Autodesk Fusion 360 part; units mm, degrees
(part 2 of 3)
extrude "Estrusione_Slitta_SG90_Sinistra_guida_01" add sketch "Schizzo30 (2)" along normal blind 23.5 bodies 11 in component "04_Torretta_parte_fissa_azimut"
ref_plane "Piano di lavoro17" through (-63.5, 0, 0) normal (1, 0, 0) x (0, 1, 0) in component "04_Torretta_parte_fissa_azimut"
sketch "Schizzo31 (2)" plane through (-63.5, 0, 0) normal (1, 0, 0) x (0, 0, -1) in component "04_Torretta_parte_fissa_azimut"
  line L0 (-74.9, 11) -> (-88.1, 11)
  line L1 (-88.1, 11) -> (-88.1, 13.5)
  line L2 (-88.1, 13.5) -> (-74.9, 13.5)
  line L3 (-74.9, 13.5) -> (-74.9, 11)
extrude "Estrusione_Slitta_SG90_Sinistra_guida_02" add sketch "Schizzo31 (2)" along normal blind 23.5 bodies 11 in component "04_Torretta_parte_fissa_azimut"
ref_plane "Piano di lavoro18" through (-63.5, 0, 0) normal (1, 0, 0) x (0, 1, 0) in component "04_Torretta_parte_fissa_azimut"
sketch "Schizzo32 (2)" plane through (-63.5, 0, 0) normal (1, 0, 0) x (0, 0, -1) in component "04_Torretta_parte_fissa_azimut"
  circle A0 centre (-81.5, -23.55) radius 1.1
extrude "Preforo_M2_5_slitta_Sinistra_01" cut sketch "Schizzo32 (2)" along normal blind 23.5 bodies 11 in component "04_Torretta_parte_fissa_azimut"
ref_plane "Piano di lavoro19" through (-63.5, 0, 0) normal (1, 0, 0) x (0, 1, 0) in component "04_Torretta_parte_fissa_azimut"
sketch "Schizzo33 (2)" plane through (-63.5, 0, 0) normal (1, 0, 0) x (0, 0, -1) in component "04_Torretta_parte_fissa_azimut"
  circle A0 centre (-81.5, 12.25) radius 1.1
extrude "Preforo_M2_5_slitta_Sinistra_02" cut sketch "Schizzo33 (2)" along normal blind 23.5 bodies 11 in component "04_Torretta_parte_fissa_azimut"
ref_plane "Piano di lavoro20" through (0, 0, 72.4) normal (0, 0, 1) x (1, 0, 0) in component "04_Torretta_parte_fissa_azimut"
sketch "Schizzo34 (2)" plane through (0, 0, 72.4) normal (0, 0, 1) x (1, 0, 0) in component "04_Torretta_parte_fissa_azimut"
  line L0 (40, -24.8) -> (63.5, -24.8)
  line L1 (63.5, -24.8) -> (63.5, 13.5)
  line L2 (63.5, 13.5) -> (40, 13.5)
  line L3 (40, 13.5) -> (40, -24.8)
extrude "Estrusione_Slitta_SG90_Destra_ripiano_Inferiore" add sketch "Schizzo34 (2)" along normal blind 2.5 bodies 11 in component "04_Torretta_parte_fissa_azimut"
ref_plane "Piano di lavoro21" through (0, 0, 88.1) normal (0, 0, 1) x (1, 0, 0) in component "04_Torretta_parte_fissa_azimut"
sketch "Schizzo35 (2)" plane through (0, 0, 88.1) normal (0, 0, 1) x (1, 0, 0) in component "04_Torretta_parte_fissa_azimut"
  line L0 (40, -24.8) -> (63.5, -24.8)
  line L1 (63.5, -24.8) -> (63.5, 13.5)
  line L2 (63.5, 13.5) -> (40, 13.5)
  line L3 (40, 13.5) -> (40, -24.8)
extrude "Estrusione_Slitta_SG90_Destra_ripiano_Superiore" add sketch "Schizzo35 (2)" along normal blind 2.5 bodies 11 in component "04_Torretta_parte_fissa_azimut"
ref_plane "Piano di lavoro22" through (0, 0, 72.4) normal (0, 0, 1) x (1, 0, 0) in component "04_Torretta_parte_fissa_azimut"
sketch "Schizzo36 (2)" plane through (0, 0, 72.4) normal (0, 0, 1) x (1, 0, 0) in component "04_Torretta_parte_fissa_azimut"
  line L0 (61.5, -8.15) -> (63.5, -8.15)
  line L1 (63.5, -8.15) -> (63.5, -3.15)
  line L2 (63.5, -3.15) -> (61.5, -3.15)
  line L3 (61.5, -3.15) -> (61.5, -8.15)
extrude "Uscita_cavo_5x2_SG90_Destra" cut sketch "Schizzo36 (2)" along normal blind 2.5 bodies 11 in component "04_Torretta_parte_fissa_azimut"
ref_plane "Piano di lavoro23" through (40, 0, 0) normal (1, 0, 0) x (0, 1, 0) in component "04_Torretta_parte_fissa_azimut"
sketch "Schizzo37 (2)" plane through (40, 0, 0) normal (1, 0, 0) x (0, 0, -1) in component "04_Torretta_parte_fissa_azimut"
  line L0 (-74.9, -24.8) -> (-88.1, -24.8)
  line L1 (-88.1, -24.8) -> (-88.1, -22.3)
  line L2 (-88.1, -22.3) -> (-74.9, -22.3)
  line L3 (-74.9, -22.3) -> (-74.9, -24.8)
extrude "Estrusione_Slitta_SG90_Destra_guida_01" add sketch "Schizzo37 (2)" along normal blind 23.5 bodies 11 in component "04_Torretta_parte_fissa_azimut"
ref_plane "Piano di lavoro24" through (40, 0, 0) normal (1, 0, 0) x (0, 1, 0) in component "04_Torretta_parte_fissa_azimut"
sketch "Schizzo38 (2)" plane through (40, 0, 0) normal (1, 0, 0) x (0, 0, -1) in component "04_Torretta_parte_fissa_azimut"
  line L0 (-74.9, 11) -> (-88.1, 11)
  line L1 (-88.1, 11) -> (-88.1, 13.5)
  line L2 (-88.1, 13.5) -> (-74.9, 13.5)
  line L3 (-74.9, 13.5) -> (-74.9, 11)
extrude "Estrusione_Slitta_SG90_Destra_guida_02" add sketch "Schizzo38 (2)" along normal blind 23.5 bodies 11 in component "04_Torretta_parte_fissa_azimut"
ref_plane "Piano di lavoro25" through (40, 0, 0) normal (1, 0, 0) x (0, 1, 0) in component "04_Torretta_parte_fissa_azimut"
sketch "Schizzo39 (2)" plane through (40, 0, 0) normal (1, 0, 0) x (0, 0, -1) in component "04_Torretta_parte_fissa_azimut"
  circle A0 centre (-81.5, -23.55) radius 1.1
extrude "Preforo_M2_5_slitta_Destra_01" cut sketch "Schizzo39 (2)" along normal blind 23.5 bodies 11 in component "04_Torretta_parte_fissa_azimut"
ref_plane "Piano di lavoro26" through (40, 0, 0) normal (1, 0, 0) x (0, 1, 0) in component "04_Torretta_parte_fissa_azimut"
sketch "Schizzo40 (2)" plane through (40, 0, 0) normal (1, 0, 0) x (0, 0, -1) in component "04_Torretta_parte_fissa_azimut"
  circle A0 centre (-81.5, 12.25) radius 1.1
extrude "Preforo_M2_5_slitta_Destra_02" cut sketch "Schizzo40 (2)" along normal blind 23.5 bodies 11 in component "04_Torretta_parte_fissa_azimut"
ref_plane "Piano di lavoro1" through (-63, 0, 0) normal (1, 0, 0) x (0, 1, 0) in component "05_Servo_TowerPro_SG90_Sinistro_statore_riferimento"
sketch "Schizzo1 (11)" plane through (-63, 0, 0) normal (1, 0, 0) x (0, 0, -1) in component "05_Servo_TowerPro_SG90_Sinistro_statore_riferimento"
  line L0 (-75.4, -17) -> (-87.6, -17)
  line L1 (-87.6, -17) -> (-87.6, 5.7)
  line L2 (-87.6, 5.7) -> (-75.4, 5.7)
  line L3 (-75.4, 5.7) -> (-75.4, -17)
extrude "Estrusione_Corpo_SG90_Sinistro" add sketch "Schizzo1 (11)" along normal blind 27 separate body makes body 12 in component "05_Servo_TowerPro_SG90_Sinistro_statore_riferimento"
ref_plane "Piano di lavoro2" through (-42, 0, 0) normal (1, 0, 0) x (0, 1, 0) in component "05_Servo_TowerPro_SG90_Sinistro_statore_riferimento"
sketch "Schizzo2 (10)" plane through (-42, 0, 0) normal (1, 0, 0) x (0, 0, -1) in component "05_Servo_TowerPro_SG90_Sinistro_statore_riferimento"
  line L0 (-75.4, -21.8) -> (-87.6, -21.8)
  line L1 (-87.6, -21.8) -> (-87.6, 10.5)
  line L2 (-87.6, 10.5) -> (-75.4, 10.5)
  line L3 (-75.4, 10.5) -> (-75.4, -21.8)
extrude "Estrusione_Alette_fissaggio_reali_SG90_Sinistro" add sketch "Schizzo2 (10)" along normal blind 2 bodies 12 in component "05_Servo_TowerPro_SG90_Sinistro_statore_riferimento"
ref_plane "Piano di lavoro3" through (-42, 0, 0) normal (1, 0, 0) x (0, 1, 0) in component "05_Servo_TowerPro_SG90_Sinistro_statore_riferimento"
sketch "Schizzo3 (9)" plane through (-42, 0, 0) normal (1, 0, 0) x (0, 0, -1) in component "05_Servo_TowerPro_SG90_Sinistro_statore_riferimento"
  circle A0 centre (-81.5, -20.05) radius 1.25
extrude "Foro_M2_5_aletta_reale_Sinistro_01" cut sketch "Schizzo3 (9)" along normal blind 2 bodies 12 in component "05_Servo_TowerPro_SG90_Sinistro_statore_riferimento"
ref_plane "Piano di lavoro4" through (-42, 0, 0) normal (1, 0, 0) x (0, 1, 0) in component "05_Servo_TowerPro_SG90_Sinistro_statore_riferimento"
sketch "Schizzo4 (8)" plane through (-42, 0, 0) normal (1, 0, 0) x (0, 0, -1) in component "05_Servo_TowerPro_SG90_Sinistro_statore_riferimento"
  circle A0 centre (-81.5, 8.75) radius 1.25
extrude "Foro_M2_5_aletta_reale_Sinistro_02" cut sketch "Schizzo4 (8)" along normal blind 2 bodies 12 in component "05_Servo_TowerPro_SG90_Sinistro_statore_riferimento"
ref_plane "Piano di lavoro1" through (36, 0, 0) normal (1, 0, 0) x (0, 1, 0) in component "06_Servo_TowerPro_SG90_Destro_statore_riferimento"
sketch "Schizzo1 (12)" plane through (36, 0, 0) normal (1, 0, 0) x (0, 0, -1) in component "06_Servo_TowerPro_SG90_Destro_statore_riferimento"
  line L0 (-75.4, -17) -> (-87.6, -17)
  line L1 (-87.6, -17) -> (-87.6, 5.7)
  line L2 (-87.6, 5.7) -> (-75.4, 5.7)
  line L3 (-75.4, 5.7) -> (-75.4, -17)
extrude "Estrusione_Corpo_SG90_Destro" add sketch "Schizzo1 (12)" along normal blind 27 separate body makes body 13 in component "06_Servo_TowerPro_SG90_Destro_statore_riferimento"
ref_plane "Piano di lavoro2" through (40, 0, 0) normal (1, 0, 0) x (0, 1, 0) in component "06_Servo_TowerPro_SG90_Destro_statore_riferimento"
sketch "Schizzo2 (11)" plane through (40, 0, 0) normal (1, 0, 0) x (0, 0, -1) in component "06_Servo_TowerPro_SG90_Destro_statore_riferimento"
  line L0 (-75.4, -21.8) -> (-87.6, -21.8)
  line L1 (-87.6, -21.8) -> (-87.6, 10.5)
  line L2 (-87.6, 10.5) -> (-75.4, 10.5)
  line L3 (-75.4, 10.5) -> (-75.4, -21.8)
extrude "Estrusione_Alette_fissaggio_reali_SG90_Destro" add sketch "Schizzo2 (11)" along normal blind 2 bodies 13 in component "06_Servo_TowerPro_SG90_Destro_statore_riferimento"
ref_plane "Piano di lavoro3" through (40, 0, 0) normal (1, 0, 0) x (0, 1, 0) in component "06_Servo_TowerPro_SG90_Destro_statore_riferimento"
sketch "Schizzo3 (10)" plane through (40, 0, 0) normal (1, 0, 0) x (0, 0, -1) in component "06_Servo_TowerPro_SG90_Destro_statore_riferimento"
  circle A0 centre (-81.5, -20.05) radius 1.25
extrude "Foro_M2_5_aletta_reale_Destro_01" cut sketch "Schizzo3 (10)" along normal blind 2 bodies 13 in component "06_Servo_TowerPro_SG90_Destro_statore_riferimento"
ref_plane "Piano di lavoro4" through (40, 0, 0) normal (1, 0, 0) x (0, 1, 0) in component "06_Servo_TowerPro_SG90_Destro_statore_riferimento"
sketch "Schizzo4 (9)" plane through (40, 0, 0) normal (1, 0, 0) x (0, 0, -1) in component "06_Servo_TowerPro_SG90_Destro_statore_riferimento"
  circle A0 centre (-81.5, 8.75) radius 1.25
extrude "Foro_M2_5_aletta_reale_Destro_02" cut sketch "Schizzo4 (9)" along normal blind 2 bodies 13 in component "06_Servo_TowerPro_SG90_Destro_statore_riferimento"
ref_plane "Piano di lavoro1" through (0, 0, 79.5) normal (0, 0, 1) x (1, 0, 0) in component "09_Torretta_parte_mobile_elevazione"
sketch "Schizzo1 (13)" plane through (0, 0, 79.5) normal (0, 0, 1) x (1, 0, 0) in component "09_Torretta_parte_mobile_elevazione"
  line L0 (-27, -20) -> (27, -20)
  line L1 (27, -20) -> (27, 50)
  line L2 (27, 50) -> (-27, 50)
  line L3 (-27, 50) -> (-27, -20)
extrude "Estrusione_Piastra_culla_mobile" add sketch "Schizzo1 (13)" along normal blind 4 separate body makes body 14 in component "09_Torretta_parte_mobile_elevazione"
sketch "Schizzo2 (12)" plane through (0, 0, 79.5) normal (0, 0, 1) x (1, 0, 0) in component "09_Torretta_parte_mobile_elevazione"
  line L0 (-3, -17) -> (3, -17)
  line L1 (3, -17) -> (3, -13)
  line L2 (3, -13) -> (-3, -13)
  line L3 (-3, -13) -> (-3, -17)
extrude "Passaggio_6x4_connettore_cannone_sotto_culla" cut sketch "Schizzo2 (12)" along normal blind 4 bodies 14 in component "09_Torretta_parte_mobile_elevazione"
sketch "Schizzo3 (11)" plane through (0, 0, 79.5) normal (0, 0, 1) x (1, 0, 0) in component "09_Torretta_parte_mobile_elevazione"
  line L0 (-7, -17.5) -> (-5, -17.5)
  line L1 (-5, -17.5) -> (-5, -12.5)
  line L2 (-5, -12.5) -> (-7, -12.5)
  line L3 (-7, -12.5) -> (-7, -17.5)
extrude "Asola_fascetta_ansa_cannone_mobile_01" cut sketch "Schizzo3 (11)" along normal blind 4 bodies 14 in component "09_Torretta_parte_mobile_elevazione"
sketch "Schizzo4 (10)" plane through (0, 0, 79.5) normal (0, 0, 1) x (1, 0, 0) in component "09_Torretta_parte_mobile_elevazione"
  line L0 (5, -17.5) -> (7, -17.5)
  line L1 (7, -17.5) -> (7, -12.5)
  line L2 (7, -12.5) -> (5, -12.5)
  line L3 (5, -12.5) -> (5, -17.5)
extrude "Asola_fascetta_ansa_cannone_mobile_02" cut sketch "Schizzo4 (10)" along normal blind 4 bodies 14 in component "09_Torretta_parte_mobile_elevazione"
sketch "Schizzo5 (4)" plane through (0, 0, 79.5) normal (0, 0, 1) x (1, 0, 0) in component "09_Torretta_parte_mobile_elevazione"
  circle A0 centre (-20, -5) radius 1.75
extrude "Foro_fissaggio_PCB_cannone_01" cut sketch "Schizzo5 (4)" along normal blind 4 bodies 14 in component "09_Torretta_parte_mobile_elevazione"
sketch "Schizzo6 (4)" plane through (0, 0, 79.5) normal (0, 0, 1) x (1, 0, 0) in component "09_Torretta_parte_mobile_elevazione"
  line L0 (-17.1, -3.3257) -> (-20, -1.6514)
  line L1 (-20, -1.6514) -> (-22.9, -3.3257)
  line L2 (-22.9, -3.3257) -> (-22.9, -6.6743)
  line L3 (-22.9, -6.6743) -> (-20, -8.3486)
  line L4 (-20, -8.3486) -> (-17.1, -6.6743)
  line L5 (-17.1, -6.6743) -> (-17.1, -3.3257)
extrude "Sede_dado_M3_PCB_cannone_01" cut sketch "Schizzo6 (4)" along normal blind 2.6 bodies 14 in component "09_Torretta_parte_mobile_elevazione"
sketch "Schizzo7 (4)" plane through (0, 0, 79.5) normal (0, 0, 1) x (1, 0, 0) in component "09_Torretta_parte_mobile_elevazione"
  circle A0 centre (20, -5) radius 1.75
extrude "Foro_fissaggio_PCB_cannone_02" cut sketch "Schizzo7 (4)" along normal blind 4 bodies 14 in component "09_Torretta_parte_mobile_elevazione"
sketch "Schizzo8 (4)" plane through (0, 0, 79.5) normal (0, 0, 1) x (1, 0, 0) in component "09_Torretta_parte_mobile_elevazione"
  line L0 (22.9, -3.3257) -> (20, -1.6514)
  line L1 (20, -1.6514) -> (17.1, -3.3257)
  line L2 (17.1, -3.3257) -> (17.1, -6.6743)
  line L3 (17.1, -6.6743) -> (20, -8.3486)
  line L4 (20, -8.3486) -> (22.9, -6.6743)
  line L5 (22.9, -6.6743) -> (22.9, -3.3257)
extrude "Sede_dado_M3_PCB_cannone_02" cut sketch "Schizzo8 (4)" along normal blind 2.6 bodies 14 in component "09_Torretta_parte_mobile_elevazione"
sketch "Schizzo9 (4)" plane through (0, 0, 79.5) normal (0, 0, 1) x (1, 0, 0) in component "09_Torretta_parte_mobile_elevazione"
  circle A0 centre (-20, 35) radius 1.75
extrude "Foro_fissaggio_PCB_cannone_03" cut sketch "Schizzo9 (4)" along normal blind 4 bodies 14 in component "09_Torretta_parte_mobile_elevazione"
sketch "Schizzo10 (4)" plane through (0, 0, 79.5) normal (0, 0, 1) x (1, 0, 0) in component "09_Torretta_parte_mobile_elevazione"
  line L0 (-17.1, 36.6743) -> (-20, 38.3486)
  line L1 (-20, 38.3486) -> (-22.9, 36.6743)
  line L2 (-22.9, 36.6743) -> (-22.9, 33.3257)
  line L3 (-22.9, 33.3257) -> (-20, 31.6514)
  line L4 (-20, 31.6514) -> (-17.1, 33.3257)
  line L5 (-17.1, 33.3257) -> (-17.1, 36.6743)
extrude "Sede_dado_M3_PCB_cannone_03" cut sketch "Schizzo10 (4)" along normal blind 2.6 bodies 14 in component "09_Torretta_parte_mobile_elevazione"
sketch "Schizzo11 (4)" plane through (0, 0, 79.5) normal (0, 0, 1) x (1, 0, 0) in component "09_Torretta_parte_mobile_elevazione"
  circle A0 centre (20, 35) radius 1.75
extrude "Foro_fissaggio_PCB_cannone_04" cut sketch "Schizzo11 (4)" along normal blind 4 bodies 14 in component "09_Torretta_parte_mobile_elevazione"
sketch "Schizzo12 (4)" plane through (0, 0, 79.5) normal (0, 0, 1) x (1, 0, 0) in component "09_Torretta_parte_mobile_elevazione"
  line L0 (22.9, 36.6743) -> (20, 38.3486)
  line L1 (20, 38.3486) -> (17.1, 36.6743)
  line L2 (17.1, 36.6743) -> (17.1, 33.3257)
  line L3 (17.1, 33.3257) -> (20, 31.6514)
  line L4 (20, 31.6514) -> (22.9, 33.3257)
  line L5 (22.9, 33.3257) -> (22.9, 36.6743)
extrude "Sede_dado_M3_PCB_cannone_04" cut sketch "Schizzo12 (4)" along normal blind 2.6 bodies 14 in component "09_Torretta_parte_mobile_elevazione"
sketch "Schizzo13 (4)" plane through (0, 0, 79.5) normal (0, 0, 1) x (1, 0, 0) in component "09_Torretta_parte_mobile_elevazione"
  circle A0 centre (-22.5, -10) radius 1.1
extrude "Preforo_cieco_guancia_cornetto_Sinistra_01" cut sketch "Schizzo13 (4)" along normal blind 3 bodies 14 in component "09_Torretta_parte_mobile_elevazione"
sketch "Schizzo14 (4)" plane through (0, 0, 79.5) normal (0, 0, 1) x (1, 0, 0) in component "09_Torretta_parte_mobile_elevazione"
  circle A0 centre (-22.5, 10) radius 1.1
extrude "Preforo_cieco_guancia_cornetto_Sinistra_02" cut sketch "Schizzo14 (4)" along normal blind 3 bodies 14 in component "09_Torretta_parte_mobile_elevazione"
sketch "Schizzo15 (4)" plane through (0, 0, 79.5) normal (0, 0, 1) x (1, 0, 0) in component "09_Torretta_parte_mobile_elevazione"
  circle A0 centre (22.5, -10) radius 1.1
extrude "Preforo_cieco_guancia_cornetto_Destra_01" cut sketch "Schizzo15 (4)" along normal blind 3 bodies 14 in component "09_Torretta_parte_mobile_elevazione"
sketch "Schizzo16 (3)" plane through (0, 0, 79.5) normal (0, 0, 1) x (1, 0, 0) in component "09_Torretta_parte_mobile_elevazione"
  circle A0 centre (22.5, 10) radius 1.1
extrude "Preforo_cieco_guancia_cornetto_Destra_02" cut sketch "Schizzo16 (3)" along normal blind 3 bodies 14 in component "09_Torretta_parte_mobile_elevazione"
ref_plane "Piano di lavoro1" through (-36, 0, 0) normal (1, 0, 0) x (0, 1, 0) in component "07_Albero_e_cornetto_croce_SG90_Sinistro_riferimento"
sketch "Schizzo1 (14)" plane through (-36, 0, 0) normal (1, 0, 0) x (0, 0, -1) in component "07_Albero_e_cornetto_croce_SG90_Sinistro_riferimento"
  circle A0 centre (-81.5, 0) radius 3
extrude "Estrusione_Albero_uscita_SG90_Sinistro" add sketch "Schizzo1 (14)" along normal blind 3.3 separate body makes body 15 in component "07_Albero_e_cornetto_croce_SG90_Sinistro_riferimento"
ref_plane "Piano di lavoro2" through (-32.7, 0, 0) normal (1, 0, 0) x (0, 1, 0) in component "07_Albero_e_cornetto_croce_SG90_Sinistro_riferimento"
sketch "Schizzo2 (13)" plane through (-32.7, 0, 0) normal (1, 0, 0) x (0, 0, -1) in component "07_Albero_e_cornetto_croce_SG90_Sinistro_riferimento"
  line L0 (-79.5, -16.5) -> (-83.5, -16.5)
  line L1 (-83.5, -16.5) -> (-83.5, 16.5)
  line L2 (-83.5, 16.5) -> (-79.5, 16.5)
  line L3 (-79.5, 16.5) -> (-79.5, -16.5)
extrude "Estrusione_Cornetto_croce_orizzontale_Sinistro" add sketch "Schizzo2 (13)" along normal blind 1.5 separate body makes body 16 in component "07_Albero_e_cornetto_croce_SG90_Sinistro_riferimento"
ref_plane "Piano di lavoro3" through (-32.7, 0, 0) normal (1, 0, 0) x (0, 1, 0) in component "07_Albero_e_cornetto_croce_SG90_Sinistro_riferimento"
sketch "Schizzo3 (12)" plane through (-32.7, 0, 0) normal (1, 0, 0) x (0, 0, -1) in component "07_Albero_e_cornetto_croce_SG90_Sinistro_riferimento"
  line L0 (-65, -2) -> (-98, -2)
  line L1 (-98, -2) -> (-98, 2)
  line L2 (-98, 2) -> (-65, 2)
  line L3 (-65, 2) -> (-65, -2)
extrude "Estrusione_Cornetto_croce_verticale_Sinistro" add sketch "Schizzo3 (12)" along normal blind 1.5 bodies 15 16 in component "07_Albero_e_cornetto_croce_SG90_Sinistro_riferimento"
ref_plane "Piano di lavoro4" through (-32.7, 0, 0) normal (1, 0, 0) x (0, 1, 0) in component "07_Albero_e_cornetto_croce_SG90_Sinistro_riferimento"
sketch "Schizzo4 (11)" plane through (-32.7, 0, 0) normal (1, 0, 0) x (0, 0, -1) in component "07_Albero_e_cornetto_croce_SG90_Sinistro_riferimento"
  circle A0 centre (-81.5, 0) radius 4
extrude "Estrusione_Mozzo_cornetto_croce_Sinistro" add sketch "Schizzo4 (11)" along normal blind 1.5 bodies 15 in component "07_Albero_e_cornetto_croce_SG90_Sinistro_riferimento"
ref_plane "Piano di lavoro1" through (32.7, 0, 0) normal (1, 0, 0) x (0, 1, 0) in component "08_Albero_e_cornetto_croce_SG90_Destro_riferimento"
sketch "Schizzo1 (15)" plane through (32.7, 0, 0) normal (1, 0, 0) x (0, 0, -1) in component "08_Albero_e_cornetto_croce_SG90_Destro_riferimento"
  circle A0 centre (-81.5, 0) radius 3
extrude "Estrusione_Albero_uscita_SG90_Destro" add sketch "Schizzo1 (15)" along normal blind 3.3 separate body makes body 17 in component "08_Albero_e_cornetto_croce_SG90_Destro_riferimento"
ref_plane "Piano di lavoro2" through (31.2, 0, 0) normal (1, 0, 0) x (0, 1, 0) in component "08_Albero_e_cornetto_croce_SG90_Destro_riferimento"
sketch "Schizzo2 (14)" plane through (31.2, 0, 0) normal (1, 0, 0) x (0, 0, -1) in component "08_Albero_e_cornetto_croce_SG90_Destro_riferimento"
  line L0 (-79.5, -16.5) -> (-83.5, -16.5)
  line L1 (-83.5, -16.5) -> (-83.5, 16.5)
  line L2 (-83.5, 16.5) -> (-79.5, 16.5)
  line L3 (-79.5, 16.5) -> (-79.5, -16.5)
extrude "Estrusione_Cornetto_croce_orizzontale_Destro" add sketch "Schizzo2 (14)" along normal blind 1.5 separate body makes body 18 in component "08_Albero_e_cornetto_croce_SG90_Destro_riferimento"
ref_plane "Piano di lavoro3" through (31.2, 0, 0) normal (1, 0, 0) x (0, 1, 0) in component "08_Albero_e_cornetto_croce_SG90_Destro_riferimento"
sketch "Schizzo3 (13)" plane through (31.2, 0, 0) normal (1, 0, 0) x (0, 0, -1) in component "08_Albero_e_cornetto_croce_SG90_Destro_riferimento"
  line L0 (-65, -2) -> (-98, -2)
  line L1 (-98, -2) -> (-98, 2)
  line L2 (-98, 2) -> (-65, 2)
  line L3 (-65, 2) -> (-65, -2)
extrude "Estrusione_Cornetto_croce_verticale_Destro" add sketch "Schizzo3 (13)" along normal blind 1.5 bodies 17 18 in component "08_Albero_e_cornetto_croce_SG90_Destro_riferimento"
ref_plane "Piano di lavoro4" through (31.2, 0, 0) normal (1, 0, 0) x (0, 1, 0) in component "08_Albero_e_cornetto_croce_SG90_Destro_riferimento"
sketch "Schizzo4 (12)" plane through (31.2, 0, 0) normal (1, 0, 0) x (0, 0, -1) in component "08_Albero_e_cornetto_croce_SG90_Destro_riferimento"
  circle A0 centre (-81.5, 0) radius 4
extrude "Estrusione_Mozzo_cornetto_croce_Destro" add sketch "Schizzo4 (12)" along normal blind 1.5 bodies 17 in component "08_Albero_e_cornetto_croce_SG90_Destro_riferimento"
ref_plane "Piano di lavoro1" through (-31, 0, 0) normal (1, 0, 0) x (0, 1, 0) in component "09A_Guancia_cornetto_Sinistra_regolabile"
sketch "Schizzo1 (16)" plane through (-31, 0, 0) normal (1, 0, 0) x (0, 0, -1) in component "09A_Guancia_cornetto_Sinistra_regolabile"
  circle A0 centre (-81.5, 0) radius 17
extrude "Estrusione_Disco_pieno_cornetto_Sinistra" add sketch "Schizzo1 (16)" along normal blind 4 separate body makes body 19 in component "09A_Guancia_cornetto_Sinistra_regolabile"
ref_plane "Piano di lavoro2" through (0, 0, 76.5) normal (0, 0, 1) x (1, 0, 0) in component "09A_Guancia_cornetto_Sinistra_regolabile"
sketch "Schizzo2 (15)" plane through (0, 0, 76.5) normal (0, 0, 1) x (1, 0, 0) in component "09A_Guancia_cornetto_Sinistra_regolabile"
  line L0 (-31, -15) -> (-18, -15)
  line L1 (-18, -15) -> (-18, 15)
  line L2 (-18, 15) -> (-31, 15)
  line L3 (-31, 15) -> (-31, -15)
extrude "Estrusione_Mensola_sotto_culla_Sinistra" add sketch "Schizzo2 (15)" along normal blind 3 separate body makes body 20 in component "09A_Guancia_cornetto_Sinistra_regolabile"
combine "Unione_disco_mensola_guancia_Sinistra" operation add target body 19 tool bodies 20 in component "09A_Guancia_cornetto_Sinistra_regolabile"
ref_plane "Piano di lavoro3" through (-31, 0, 0) normal (1, 0, 0) x (0, 1, 0) in component "09A_Guancia_cornetto_Sinistra_regolabile"
sketch "Schizzo3 (14)" plane through (-31, 0, 0) normal (1, 0, 0) x (0, 0, -1) in component "09A_Guancia_cornetto_Sinistra_regolabile"
  circle A0 centre (-81.5, 0) radius 5
extrude "Accesso_vite_centrale_cornetto_Sinistra" cut sketch "Schizzo3 (14)" along normal blind 4 bodies 19 in component "09A_Guancia_cornetto_Sinistra_regolabile"
ref_plane "Piano di lavoro4" through (0, 0, 76.5) normal (0, 0, 1) x (1, 0, 0) in component "09A_Guancia_cornetto_Sinistra_regolabile"
sketch "Schizzo4 (13)" plane through (0, 0, 76.5) normal (0, 0, 1) x (1, 0, 0) in component "09A_Guancia_cornetto_Sinistra_regolabile"
  line L0 (-25, -11.45) -> (-20, -11.45)
  line L1 (-20, -11.45) -> (-20, -8.55)
  line L2 (-20, -8.55) -> (-25, -8.55)
  line L3 (-25, -8.55) -> (-25, -11.45)
extrude "Asola_regolazione_guancia_Sinistra_01" cut sketch "Schizzo4 (13)" along normal blind 3 bodies 19 in component "09A_Guancia_cornetto_Sinistra_regolabile"
ref_plane "Piano di lavoro5" through (0, 0, 76.5) normal (0, 0, 1) x (1, 0, 0) in component "09A_Guancia_cornetto_Sinistra_regolabile"
sketch "Schizzo5 (5)" plane through (0, 0, 76.5) normal (0, 0, 1) x (1, 0, 0) in component "09A_Guancia_cornetto_Sinistra_regolabile"
  line L0 (-25, 8.55) -> (-20, 8.55)
  line L1 (-20, 8.55) -> (-20, 11.45)
  line L2 (-20, 11.45) -> (-25, 11.45)
  line L3 (-25, 11.45) -> (-25, 8.55)
extrude "Asola_regolazione_guancia_Sinistra_02" cut sketch "Schizzo5 (5)" along normal blind 3 bodies 19 in component "09A_Guancia_cornetto_Sinistra_regolabile"
ref_plane "Piano di lavoro1" through (27, 0, 0) normal (1, 0, 0) x (0, 1, 0) in component "09B_Guancia_cornetto_Destra_regolabile"
sketch "Schizzo1 (17)" plane through (27, 0, 0) normal (1, 0, 0) x (0, 0, -1) in component "09B_Guancia_cornetto_Destra_regolabile"
  circle A0 centre (-81.5, 0) radius 17
extrude "Estrusione_Disco_pieno_cornetto_Destra" add sketch "Schizzo1 (17)" along normal blind 4 separate body makes body 21 in component "09B_Guancia_cornetto_Destra_regolabile"
ref_plane "Piano di lavoro2" through (0, 0, 76.5) normal (0, 0, 1) x (1, 0, 0) in component "09B_Guancia_cornetto_Destra_regolabile"
sketch "Schizzo2 (16)" plane through (0, 0, 76.5) normal (0, 0, 1) x (1, 0, 0) in component "09B_Guancia_cornetto_Destra_regolabile"
  line L0 (18, -15) -> (31, -15)
  line L1 (31, -15) -> (31, 15)
  line L2 (31, 15) -> (18, 15)
  line L3 (18, 15) -> (18, -15)
extrude "Estrusione_Mensola_sotto_culla_Destra" add sketch "Schizzo2 (16)" along normal blind 3 separate body makes body 22 in component "09B_Guancia_cornetto_Destra_regolabile"
combine "Unione_disco_mensola_guancia_Destra" operation add target body 21 tool bodies 22 in component "09B_Guancia_cornetto_Destra_regolabile"
ref_plane "Piano di lavoro3" through (27, 0, 0) normal (1, 0, 0) x (0, 1, 0) in component "09B_Guancia_cornetto_Destra_regolabile"
sketch "Schizzo3 (15)" plane through (27, 0, 0) normal (1, 0, 0) x (0, 0, -1) in component "09B_Guancia_cornetto_Destra_regolabile"
  circle A0 centre (-81.5, 0) radius 5
extrude "Accesso_vite_centrale_cornetto_Destra" cut sketch "Schizzo3 (15)" along normal blind 4 bodies 21 in component "09B_Guancia_cornetto_Destra_regolabile"
ref_plane "Piano di lavoro4" through (0, 0, 76.5) normal (0, 0, 1) x (1, 0, 0) in component "09B_Guancia_cornetto_Destra_regolabile"
sketch "Schizzo4 (14)" plane through (0, 0, 76.5) normal (0, 0, 1) x (1, 0, 0) in component "09B_Guancia_cornetto_Destra_regolabile"
  line L0 (20, -11.45) -> (25, -11.45)
  line L1 (25, -11.45) -> (25, -8.55)
  line L2 (25, -8.55) -> (20, -8.55)
  line L3 (20, -8.55) -> (20, -11.45)
extrude "Asola_regolazione_guancia_Destra_01" cut sketch "Schizzo4 (14)" along normal blind 3 bodies 21 in component "09B_Guancia_cornetto_Destra_regolabile"
ref_plane "Piano di lavoro5" through (0, 0, 76.5) normal (0, 0, 1) x (1, 0, 0) in component "09B_Guancia_cornetto_Destra_regolabile"
sketch "Schizzo5 (6)" plane through (0, 0, 76.5) normal (0, 0, 1) x (1, 0, 0) in component "09B_Guancia_cornetto_Destra_regolabile"
  line L0 (20, 8.55) -> (25, 8.55)
  line L1 (25, 8.55) -> (25, 11.45)
  line L2 (25, 11.45) -> (20, 11.45)
  line L3 (20, 11.45) -> (20, 8.55)
extrude "Asola_regolazione_guancia_Destra_02" cut sketch "Schizzo5 (6)" along normal blind 3 bodies 21 in component "09B_Guancia_cornetto_Destra_regolabile"
ref_plane "Piano di lavoro1" through (0, 0, 83.5) normal (0, 0, 1) x (1, 0, 0) in component "10_Modulo_cannone_reale_PCB_solenoide_canna"
sketch "Schizzo1 (18)" plane through (0, 0, 83.5) normal (0, 0, 1) x (1, 0, 0) in component "10_Modulo_cannone_reale_PCB_solenoide_canna"
  line L0 (-25, -10) -> (25, -10)
  line L1 (25, -10) -> (25, 40)
  line L2 (25, 40) -> (-25, 40)
  line L3 (-25, 40) -> (-25, -10)
extrude "Estrusione_PCB_modulo_cannone_50x50" add sketch "Schizzo1 (18)" along normal blind 2 separate body makes body 23 in component "10_Modulo_cannone_reale_PCB_solenoide_canna"
sketch "Schizzo2 (17)" plane through (0, 0, 83.5) normal (0, 0, 1) x (1, 0, 0) in component "10_Modulo_cannone_reale_PCB_solenoide_canna"
  circle A0 centre (-20, -5) radius 1.75
extrude "Foro_PCB_reale_01" cut sketch "Schizzo2 (17)" along normal blind 2 bodies 23 in component "10_Modulo_cannone_reale_PCB_solenoide_canna"
sketch "Schizzo3 (16)" plane through (0, 0, 83.5) normal (0, 0, 1) x (1, 0, 0) in component "10_Modulo_cannone_reale_PCB_solenoide_canna"
  circle A0 centre (20, -5) radius 1.75
extrude "Foro_PCB_reale_02" cut sketch "Schizzo3 (16)" along normal blind 2 bodies 23 in component "10_Modulo_cannone_reale_PCB_solenoide_canna"
sketch "Schizzo4 (15)" plane through (0, 0, 83.5) normal (0, 0, 1) x (1, 0, 0) in component "10_Modulo_cannone_reale_PCB_solenoide_canna"
  circle A0 centre (-20, 35) radius 1.75
extrude "Foro_PCB_reale_03" cut sketch "Schizzo4 (15)" along normal blind 2 bodies 23 in component "10_Modulo_cannone_reale_PCB_solenoide_canna"
sketch "Schizzo5 (7)" plane through (0, 0, 83.5) normal (0, 0, 1) x (1, 0, 0) in component "10_Modulo_cannone_reale_PCB_solenoide_canna"
  circle A0 centre (20, 35) radius 1.75
extrude "Foro_PCB_reale_04" cut sketch "Schizzo5 (7)" along normal blind 2 bodies 23 in component "10_Modulo_cannone_reale_PCB_solenoide_canna"
ref_plane "Piano di lavoro2" through (0, 0, 85.5) normal (0, 0, 1) x (1, 0, 0) in component "10_Modulo_cannone_reale_PCB_solenoide_canna"
sketch "Schizzo6 (5)" plane through (0, 0, 85.5) normal (0, 0, 1) x (1, 0, 0) in component "10_Modulo_cannone_reale_PCB_solenoide_canna"
  line L0 (-10, 2.5) -> (10, 2.5)
  line L1 (10, 2.5) -> (10, 27.5)
  line L2 (10, 27.5) -> (-10, 27.5)
  line L3 (-10, 27.5) -> (-10, 2.5)
extrude "Estrusione_Appoggio_solenoide_su_PCB" add sketch "Schizzo6 (5)" along normal blind 1 separate body makes body 24 in component "10_Modulo_cannone_reale_PCB_solenoide_canna"
ref_plane "Piano di lavoro3" through (0, 2.5, 0) normal (0, 1, 0) x (0, 0, 1) in component "10_Modulo_cannone_reale_PCB_solenoide_canna"
sketch "Schizzo7 (5)" plane through (0, 2.5, 0) normal (0, 1, 0) x (1, 0, 0) in component "10_Modulo_cannone_reale_PCB_solenoide_canna"
  circle A0 centre (0, -96.5) radius 10
extrude "Estrusione_Corpo_solenoide_riferimento" add sketch "Schizzo7 (5)" along normal blind 25 separate body makes body 25 in component "10_Modulo_cannone_reale_PCB_solenoide_canna"
ref_plane "Piano di lavoro4" through (0, 2.5, 0) normal (0, 1, 0) x (0, 0, 1) in component "10_Modulo_cannone_reale_PCB_solenoide_canna"
sketch "Schizzo8 (5)" plane through (0, 2.5, 0) normal (0, 1, 0) x (1, 0, 0) in component "10_Modulo_cannone_reale_PCB_solenoide_canna"
  circle A0 centre (0, -96.5) radius 5
extrude "Passaggio_canna_nel_solenoide" cut sketch "Schizzo8 (5)" along normal blind 25 bodies 25 in component "10_Modulo_cannone_reale_PCB_solenoide_canna"
ref_plane "Piano di lavoro5" through (0, 27.5, 0) normal (0, 1, 0) x (0, 0, 1) in component "10_Modulo_cannone_reale_PCB_solenoide_canna"
sketch "Schizzo9 (5)" plane through (0, 27.5, 0) normal (0, 1, 0) x (1, 0, 0) in component "10_Modulo_cannone_reale_PCB_solenoide_canna"
  circle A0 centre (0, -96.5) radius 5
extrude "Estrusione_Canna_tubolare_esterna" add sketch "Schizzo9 (5)" along normal blind 46 separate body makes body 26 in component "10_Modulo_cannone_reale_PCB_solenoide_canna"
ref_plane "Piano di lavoro6" through (0, 27.5, 0) normal (0, 1, 0) x (0, 0, 1) in component "10_Modulo_cannone_reale_PCB_solenoide_canna"
sketch "Schizzo10 (5)" plane through (0, 27.5, 0) normal (0, 1, 0) x (1, 0, 0) in component "10_Modulo_cannone_reale_PCB_solenoide_canna"
  circle A0 centre (0, -96.5) radius 4
extrude "Foro_interno_canna_tubolare" cut sketch "Schizzo10 (5)" along normal blind 46 bodies 26 in component "10_Modulo_cannone_reale_PCB_solenoide_canna"
ref_plane "Piano di lavoro1" through (0, -38, 0) normal (0, 1, 0) x (0, 0, 1) in component "11_Guscio_fisso_posteriore_torretta_removibile"
sketch "Schizzo1 (19)" plane through (0, -38, 0) normal (0, 1, 0) x (1, 0, 0) in component "11_Guscio_fisso_posteriore_torretta_removibile"
  line L0 (-43, -49.5) -> (43, -49.5)
  line L1 (43, -49.5) -> (43, -102.5)
  line L2 (43, -102.5) -> (-43, -102.5)
  line L3 (-43, -102.5) -> (-43, -49.5)
extrude "Estrusione_Parete_posteriore_guscio_torretta" add sketch "Schizzo1 (19)" along normal blind 2.5 separate body makes body 27 in component "11_Guscio_fisso_posteriore_torretta_removibile"
ref_plane "Piano di lavoro2" through (-43, 0, 0) normal (1, 0, 0) x (0, 1, 0) in component "11_Guscio_fisso_posteriore_torretta_removibile"
sketch "Schizzo2 (18)" plane through (-43, 0, 0) normal (1, 0, 0) x (0, 0, -1) in component "11_Guscio_fisso_posteriore_torretta_removibile"
  line L0 (-49.5, -38) -> (-102.5, -38)
  line L1 (-102.5, -38) -> (-102.5, -27.8)
  line L2 (-102.5, -27.8) -> (-49.5, -27.8)
  line L3 (-49.5, -27.8) -> (-49.5, -38)
extrude "Estrusione_Fianco_cofano_Sinistra" add sketch "Schizzo2 (18)" along normal blind 2.5 bodies 27 in component "11_Guscio_fisso_posteriore_torretta_removibile"
ref_plane "Piano di lavoro3" through (40.5, 0, 0) normal (1, 0, 0) x (0, 1, 0) in component "11_Guscio_fisso_posteriore_torretta_removibile"
sketch "Schizzo3 (17)" plane through (40.5, 0, 0) normal (1, 0, 0) x (0, 0, -1) in component "11_Guscio_fisso_posteriore_torretta_removibile"
  line L0 (-49.5, -38) -> (-102.5, -38)
  line L1 (-102.5, -38) -> (-102.5, -27.8)
  line L2 (-102.5, -27.8) -> (-49.5, -27.8)
  line L3 (-49.5, -27.8) -> (-49.5, -38)
extrude "Estrusione_Fianco_cofano_Destra" add sketch "Schizzo3 (17)" along normal blind 2.5 bodies 27 in component "11_Guscio_fisso_posteriore_torretta_removibile"
ref_plane "Piano di lavoro4" through (0, 0, 100) normal (0, 0, 1) x (1, 0, 0) in component "11_Guscio_fisso_posteriore_torretta_removibile"
sketch "Schizzo4 (16)" plane through (0, 0, 100) normal (0, 0, 1) x (1, 0, 0) in component "11_Guscio_fisso_posteriore_torretta_removibile"
  line L0 (-43, -38) -> (43, -38)
  line L1 (43, -38) -> (43, -27.8)
  line L2 (43, -27.8) -> (-43, -27.8)
  line L3 (-43, -27.8) -> (-43, -38)
extrude "Estrusione_Tetto_cofano_posteriore" add sketch "Schizzo4 (16)" along normal blind 2.5 bodies 27 in component "11_Guscio_fisso_posteriore_torretta_removibile"
ref_plane "Piano di lavoro5" through (-43, 0, 0) normal (1, 0, 0) x (0, 1, 0) in component "11_Guscio_fisso_posteriore_torretta_removibile"
sketch "Schizzo5 (8)" plane through (-43, 0, 0) normal (1, 0, 0) x (0, 0, -1) in component "11_Guscio_fisso_posteriore_torretta_removibile"
  circle A0 centre (-54.5, -30.3) radius 1.35
extrude "Foro_M2_5_cofano_Sinistra_01" cut sketch "Schizzo5 (8)" along normal blind 2.5 bodies 27 in component "11_Guscio_fisso_posteriore_torretta_removibile"
ref_plane "Piano di lavoro27" through (-40, 0, 0) normal (1, 0, 0) x (0, 1, 0) in component "04_Torretta_parte_fissa_azimut"
sketch "Schizzo41 (2)" plane through (-40, 0, 0) normal (1, 0, 0) x (0, 0, -1) in component "04_Torretta_parte_fissa_azimut"
  circle A0 centre (-54.5, -30.3) radius 1.1
extrude "Preforo_M2_5_cofano_telaio_Sinistra_01" cut sketch "Schizzo41 (2)" along normal blind 4 bodies 11 in component "04_Torretta_parte_fissa_azimut"
ref_plane "Piano di lavoro6" through (-43, 0, 0) normal (1, 0, 0) x (0, 1, 0) in component "11_Guscio_fisso_posteriore_torretta_removibile"
sketch "Schizzo6 (6)" plane through (-43, 0, 0) normal (1, 0, 0) x (0, 0, -1) in component "11_Guscio_fisso_posteriore_torretta_removibile"
  circle A0 centre (-94.5, -30.3) radius 1.35
extrude "Foro_M2_5_cofano_Sinistra_02" cut sketch "Schizzo6 (6)" along normal blind 2.5 bodies 27 in component "11_Guscio_fisso_posteriore_torretta_removibile"
ref_plane "Piano di lavoro28" through (-40, 0, 0) normal (1, 0, 0) x (0, 1, 0) in component "04_Torretta_parte_fissa_azimut"
sketch "Schizzo42 (2)" plane through (-40, 0, 0) normal (1, 0, 0) x (0, 0, -1) in component "04_Torretta_parte_fissa_azimut"
  circle A0 centre (-94.5, -30.3) radius 1.1
extrude "Preforo_M2_5_cofano_telaio_Sinistra_02" cut sketch "Schizzo42 (2)" along normal blind 4 bodies 11 in component "04_Torretta_parte_fissa_azimut"
ref_plane "Piano di lavoro7" through (40.5, 0, 0) normal (1, 0, 0) x (0, 1, 0) in component "11_Guscio_fisso_posteriore_torretta_removibile"
sketch "Schizzo7 (6)" plane through (40.5, 0, 0) normal (1, 0, 0) x (0, 0, -1) in component "11_Guscio_fisso_posteriore_torretta_removibile"
  circle A0 centre (-54.5, -30.3) radius 1.35
extrude "Foro_M2_5_cofano_Destra_01" cut sketch "Schizzo7 (6)" along normal blind 2.5 bodies 27 in component "11_Guscio_fisso_posteriore_torretta_removibile"
ref_plane "Piano di lavoro29" through (36, 0, 0) normal (1, 0, 0) x (0, 1, 0) in component "04_Torretta_parte_fissa_azimut"
sketch "Schizzo43 (2)" plane through (36, 0, 0) normal (1, 0, 0) x (0, 0, -1) in component "04_Torretta_parte_fissa_azimut"
  circle A0 centre (-54.5, -30.3) radius 1.1
extrude "Preforo_M2_5_cofano_telaio_Destra_01" cut sketch "Schizzo43 (2)" along normal blind 4 bodies 11 in component "04_Torretta_parte_fissa_azimut"
ref_plane "Piano di lavoro8" through (40.5, 0, 0) normal (1, 0, 0) x (0, 1, 0) in component "11_Guscio_fisso_posteriore_torretta_removibile"
sketch "Schizzo8 (6)" plane through (40.5, 0, 0) normal (1, 0, 0) x (0, 0, -1) in component "11_Guscio_fisso_posteriore_torretta_removibile"
  circle A0 centre (-94.5, -30.3) radius 1.35
extrude "Foro_M2_5_cofano_Destra_02" cut sketch "Schizzo8 (6)" along normal blind 2.5 bodies 27 in component "11_Guscio_fisso_posteriore_torretta_removibile"
ref_plane "Piano di lavoro30" through (36, 0, 0) normal (1, 0, 0) x (0, 1, 0) in component "04_Torretta_parte_fissa_azimut"
sketch "Schizzo44" plane through (36, 0, 0) normal (1, 0, 0) x (0, 0, -1) in component "04_Torretta_parte_fissa_azimut"
  circle A0 centre (-94.5, -30.3) radius 1.1
extrude "Preforo_M2_5_cofano_telaio_Destra_02" cut sketch "Schizzo44" along normal blind 4 bodies 11 in component "04_Torretta_parte_fissa_azimut"
ref_plane "Piano di lavoro1" through (-66.5, 0, 0) normal (1, 0, 0) x (0, 1, 0) in component "12_Carter_SG90_Sinistro_removibile"
sketch "Schizzo1 (20)" plane through (-66.5, 0, 0) normal (1, 0, 0) x (0, 0, -1) in component "12_Carter_SG90_Sinistro_removibile"
  line L0 (-71.9, -27.8) -> (-93.6, -27.8)
  line L1 (-93.6, -27.8) -> (-93.6, 16.5)
  line L2 (-93.6, 16.5) -> (-71.9, 16.5)
  line L3 (-71.9, 16.5) -> (-71.9, -27.8)
extrude "Estrusione_Parete_esterna_carter_Sinistro" add sketch "Schizzo1 (20)" along normal blind 2.5 separate body makes body 28 in component "12_Carter_SG90_Sinistro_removibile"
ref_plane "Piano di lavoro2" through (0, -27.8, 0) normal (0, 1, 0) x (0, 0, 1) in component "12_Carter_SG90_Sinistro_removibile"
sketch "Schizzo2 (19)" plane through (0, -27.8, 0) normal (0, 1, 0) x (1, 0, 0) in component "12_Carter_SG90_Sinistro_removibile"
  line L0 (-66.5, -71.9) -> (-40.5, -71.9)
  line L1 (-40.5, -71.9) -> (-40.5, -93.6)
  line L2 (-40.5, -93.6) -> (-66.5, -93.6)
  line L3 (-66.5, -93.6) -> (-66.5, -71.9)
extrude "Estrusione_Parete_Posteriore_carter_Sinistro" add sketch "Schizzo2 (19)" along normal blind 2.5 bodies 28 in component "12_Carter_SG90_Sinistro_removibile"
ref_plane "Piano di lavoro3" through (0, 14, 0) normal (0, 1, 0) x (0, 0, 1) in component "12_Carter_SG90_Sinistro_removibile"
sketch "Schizzo3 (18)" plane through (0, 14, 0) normal (0, 1, 0) x (1, 0, 0) in component "12_Carter_SG90_Sinistro_removibile"
  line L0 (-66.5, -71.9) -> (-40.5, -71.9)
  line L1 (-40.5, -71.9) -> (-40.5, -93.6)
  line L2 (-40.5, -93.6) -> (-66.5, -93.6)
  line L3 (-66.5, -93.6) -> (-66.5, -71.9)
extrude "Estrusione_Parete_Anteriore_carter_Sinistro" add sketch "Schizzo3 (18)" along normal blind 2.5 bodies 28 in component "12_Carter_SG90_Sinistro_removibile"
ref_plane "Piano di lavoro4" through (0, 0, 91.1) normal (0, 0, 1) x (1, 0, 0) in component "12_Carter_SG90_Sinistro_removibile"
sketch "Schizzo4 (17)" plane through (0, 0, 91.1) normal (0, 0, 1) x (1, 0, 0) in component "12_Carter_SG90_Sinistro_removibile"
  line L0 (-66.5, -27.8) -> (-40.5, -27.8)
  line L1 (-40.5, -27.8) -> (-40.5, 16.5)
  line L2 (-40.5, 16.5) -> (-66.5, 16.5)
  line L3 (-66.5, 16.5) -> (-66.5, -27.8)
extrude "Estrusione_Tetto_carter_Sinistro" add sketch "Schizzo4 (17)" along normal blind 2.5 bodies 28 in component "12_Carter_SG90_Sinistro_removibile"
ref_plane "Piano di lavoro5" through (-66.5, 0, 0) normal (1, 0, 0) x (0, 1, 0) in component "12_Carter_SG90_Sinistro_removibile"
sketch "Schizzo5 (9)" plane through (-66.5, 0, 0) normal (1, 0, 0) x (0, 0, -1) in component "12_Carter_SG90_Sinistro_removibile"
  circle A0 centre (-81.5, -23.55) radius 1.35
extrude "Foro_M2_5_carter_Sinistro_01" cut sketch "Schizzo5 (9)" along normal blind 2.5 bodies 28 in component "12_Carter_SG90_Sinistro_removibile"
ref_plane "Piano di lavoro6" through (-66.5, 0, 0) normal (1, 0, 0) x (0, 1, 0) in component "12_Carter_SG90_Sinistro_removibile"
sketch "Schizzo6 (7)" plane through (-66.5, 0, 0) normal (1, 0, 0) x (0, 0, -1) in component "12_Carter_SG90_Sinistro_removibile"
  circle A0 centre (-81.5, 12.25) radius 1.35
extrude "Foro_M2_5_carter_Sinistro_02" cut sketch "Schizzo6 (7)" along normal blind 2.5 bodies 28 in component "12_Carter_SG90_Sinistro_removibile"
ref_plane "Piano di lavoro1" through (64, 0, 0) normal (1, 0, 0) x (0, 1, 0) in component "13_Carter_SG90_Destro_removibile"
sketch "Schizzo1 (21)" plane through (64, 0, 0) normal (1, 0, 0) x (0, 0, -1) in component "13_Carter_SG90_Destro_removibile"
  line L0 (-71.9, -27.8) -> (-93.6, -27.8)
  line L1 (-93.6, -27.8) -> (-93.6, 16.5)
  line L2 (-93.6, 16.5) -> (-71.9, 16.5)
  line L3 (-71.9, 16.5) -> (-71.9, -27.8)
extrude "Estrusione_Parete_esterna_carter_Destro" add sketch "Schizzo1 (21)" along normal blind 2.5 separate body makes body 29 in component "13_Carter_SG90_Destro_removibile"
ref_plane "Piano di lavoro2" through (0, -27.8, 0) normal (0, 1, 0) x (0, 0, 1) in component "13_Carter_SG90_Destro_removibile"
sketch "Schizzo2 (20)" plane through (0, -27.8, 0) normal (0, 1, 0) x (1, 0, 0) in component "13_Carter_SG90_Destro_removibile"
  line L0 (40.5, -71.9) -> (66.5, -71.9)
  line L1 (66.5, -71.9) -> (66.5, -93.6)
  line L2 (66.5, -93.6) -> (40.5, -93.6)
  line L3 (40.5, -93.6) -> (40.5, -71.9)
extrude "Estrusione_Parete_Posteriore_carter_Destro" add sketch "Schizzo2 (20)" along normal blind 2.5 bodies 29 in component "13_Carter_SG90_Destro_removibile"
ref_plane "Piano di lavoro3" through (0, 14, 0) normal (0, 1, 0) x (0, 0, 1) in component "13_Carter_SG90_Destro_removibile"
sketch "Schizzo3 (19)" plane through (0, 14, 0) normal (0, 1, 0) x (1, 0, 0) in component "13_Carter_SG90_Destro_removibile"
  line L0 (40.5, -71.9) -> (66.5, -71.9)
  line L1 (66.5, -71.9) -> (66.5, -93.6)
  line L2 (66.5, -93.6) -> (40.5, -93.6)
  line L3 (40.5, -93.6) -> (40.5, -71.9)
extrude "Estrusione_Parete_Anteriore_carter_Destro" add sketch "Schizzo3 (19)" along normal blind 2.5 bodies 29 in component "13_Carter_SG90_Destro_removibile"
ref_plane "Piano di lavoro4" through (0, 0, 91.1) normal (0, 0, 1) x (1, 0, 0) in component "13_Carter_SG90_Destro_removibile"
sketch "Schizzo4 (18)" plane through (0, 0, 91.1) normal (0, 0, 1) x (1, 0, 0) in component "13_Carter_SG90_Destro_removibile"
  line L0 (40.5, -27.8) -> (66.5, -27.8)
  line L1 (66.5, -27.8) -> (66.5, 16.5)
  line L2 (66.5, 16.5) -> (40.5, 16.5)
  line L3 (40.5, 16.5) -> (40.5, -27.8)
extrude "Estrusione_Tetto_carter_Destro" add sketch "Schizzo4 (18)" along normal blind 2.5 bodies 29 in component "13_Carter_SG90_Destro_removibile"
ref_plane "Piano di lavoro5" through (64, 0, 0) normal (1, 0, 0) x (0, 1, 0) in component "13_Carter_SG90_Destro_removibile"
sketch "Schizzo5 (10)" plane through (64, 0, 0) normal (1, 0, 0) x (0, 0, -1) in component "13_Carter_SG90_Destro_removibile"
  circle A0 centre (-81.5, -23.55) radius 1.35
extrude "Foro_M2_5_carter_Destro_01" cut sketch "Schizzo5 (10)" along normal blind 2.5 bodies 29 in component "13_Carter_SG90_Destro_removibile"
ref_plane "Piano di lavoro6" through (64, 0, 0) normal (1, 0, 0) x (0, 1, 0) in component "13_Carter_SG90_Destro_removibile"
sketch "Schizzo6 (8)" plane through (64, 0, 0) normal (1, 0, 0) x (0, 0, -1) in component "13_Carter_SG90_Destro_removibile"
  circle A0 centre (-81.5, 12.25) radius 1.35
extrude "Foro_M2_5_carter_Destro_02" cut sketch "Schizzo6 (8)" along normal blind 2.5 bodies 29 in component "13_Carter_SG90_Destro_removibile"
ref_plane "Piano di lavoro1" through (0, 0, 83.5) normal (0, 0, 1) x (1, 0, 0) in component "14_Guscio_mobile_cannone_removibile"
sketch "Schizzo1 (22)" plane through (0, 0, 83.5) normal (0, 0, 1) x (1, 0, 0) in component "14_Guscio_mobile_cannone_removibile"
  line L0 (-28, -13) -> (-25.5, -13)
  line L1 (-25.5, -13) -> (-25.5, 43)
  line L2 (-25.5, 43) -> (-28, 43)
  line L3 (-28, 43) -> (-28, -13)
extrude "Estrusione_Parete_mobile_Ovest" add sketch "Schizzo1 (22)" along normal blind 26 separate body makes body 30 in component "14_Guscio_mobile_cannone_removibile"
sketch "Schizzo2 (21)" plane through (0, 0, 83.5) normal (0, 0, 1) x (1, 0, 0) in component "14_Guscio_mobile_cannone_removibile"
  line L0 (-28, -13) -> (28, -13)
  line L1 (28, -13) -> (28, -10.5)
  line L2 (28, -10.5) -> (-28, -10.5)
  line L3 (-28, -10.5) -> (-28, -13)
extrude "Estrusione_Parete_mobile_Posteriore" add sketch "Schizzo2 (21)" along normal blind 26 bodies 30 in component "14_Guscio_mobile_cannone_removibile"
sketch "Schizzo3 (20)" plane through (0, 0, 83.5) normal (0, 0, 1) x (1, 0, 0) in component "14_Guscio_mobile_cannone_removibile"
  line L0 (25.5, -13) -> (28, -13)
  line L1 (28, -13) -> (28, 43)
  line L2 (28, 43) -> (25.5, 43)
  line L3 (25.5, 43) -> (25.5, -13)
extrude "Estrusione_Parete_mobile_Est" add sketch "Schizzo3 (20)" along normal blind 26 bodies 30 in component "14_Guscio_mobile_cannone_removibile"
ref_plane "Piano di lavoro2" through (-28, 0, 0) normal (1, 0, 0) x (0, 1, 0) in component "14_Guscio_mobile_cannone_removibile"
sketch "Schizzo4 (19)" plane through (-28, 0, 0) normal (1, 0, 0) x (0, 0, -1) in component "14_Guscio_mobile_cannone_removibile"
  circle A0 centre (-81.5, 0) radius 17.5
extrude "Scasso_guancia_elevazione_Ovest" cut sketch "Schizzo4 (19)" along normal blind 2.5 bodies 14 in component "09_Torretta_parte_mobile_elevazione"
extrude "Estrusione6'" cut sketch "Schizzo4 (19)" along normal blind 2.5 bodies 19 makes body 31 at (-31, -1.093, 68.5819) in component "09A_Guancia_cornetto_Sinistra_regolabile"
extrude "Estrusione4" cut sketch "Schizzo4 (19)" along normal blind 2.5 bodies 30 in component "14_Guscio_mobile_cannone_removibile"
ref_plane "Piano di lavoro3" through (25.5, 0, 0) normal (1, 0, 0) x (0, 1, 0) in component "14_Guscio_mobile_cannone_removibile"
sketch "Schizzo5 (11)" plane through (25.5, 0, 0) normal (1, 0, 0) x (0, 0, -1) in component "14_Guscio_mobile_cannone_removibile"
  circle A0 centre (-81.5, 0) radius 17.5
extrude "Scasso_guancia_elevazione_Est" cut sketch "Schizzo5 (11)" along normal blind 2.5 bodies 14 in component "09_Torretta_parte_mobile_elevazione"
extrude "Estrusione6''" cut sketch "Schizzo5 (11)" along normal blind 2.5 bodies 21 makes body 32 at (23.3333, -2.85, 79.5) in component "09B_Guancia_cornetto_Destra_regolabile"
extrude "Estrusione5" cut sketch "Schizzo5 (11)" along normal blind 2.5 bodies 30 in component "14_Guscio_mobile_cannone_removibile"
ref_plane "Piano di lavoro4" through (0, 0, 107) normal (0, 0, 1) x (1, 0, 0) in component "14_Guscio_mobile_cannone_removibile"
sketch "Schizzo6 (9)" plane through (0, 0, 107) normal (0, 0, 1) x (1, 0, 0) in component "14_Guscio_mobile_cannone_removibile"
  line L0 (-28, -13) -> (28, -13)
  line L1 (28, -13) -> (28, 43)
  line L2 (28, 43) -> (-28, 43)
  line L3 (-28, 43) -> (-28, -13)
extrude "Estrusione_Tetto_guscio_mobile_cannone" add sketch "Schizzo6 (9)" along normal blind 2.5 bodies 30 in component "14_Guscio_mobile_cannone_removibile"
ref_plane "Piano di lavoro5" through (0, 0, 106.2) normal (0, 0, 1) x (1, 0, 0) in component "14_Guscio_mobile_cannone_removibile"
sketch "Schizzo7 (7)" plane through (0, 0, 106.2) normal (0, 0, 1) x (1, 0, 0) in component "14_Guscio_mobile_cannone_removibile"
  line L0 (-15, -13) -> (-7, -13)
  line L1 (-7, -13) -> (-7, 2)
  line L2 (-7, 2) -> (-15, 2)
  line L3 (-15, 2) -> (-15, -13)
extrude "Estrusione_Longherone_rinforzo_tasca_culatta_Ovest" add sketch "Schizzo7 (7)" along normal blind 1 bodies 30 in component "14_Guscio_mobile_cannone_removibile"
sketch "Schizzo8 (7)" plane through (0, 0, 106.2) normal (0, 0, 1) x (1, 0, 0) in component "14_Guscio_mobile_cannone_removibile"
  line L0 (7, -13) -> (15, -13)
  line L1 (15, -13) -> (15, 2)
  line L2 (15, 2) -> (7, 2)
  line L3 (7, 2) -> (7, -13)
extrude "Estrusione_Longherone_rinforzo_tasca_culatta_Est" add sketch "Schizzo8 (7)" along normal blind 1 bodies 30 in component "14_Guscio_mobile_cannone_removibile"
sketch "Schizzo9 (6)" plane through (0, 0, 106.2) normal (0, 0, 1) x (1, 0, 0) in component "14_Guscio_mobile_cannone_removibile"
  line L0 (-15, -1) -> (15, -1)
  line L1 (15, -1) -> (15, 2)
  line L2 (15, 2) -> (-15, 2)
  line L3 (-15, 2) -> (-15, -1)
extrude "Estrusione_Traversa_anteriore_rinforzo_tasca_culatta" add sketch "Schizzo9 (6)" along normal blind 1 bodies 30 in component "14_Guscio_mobile_cannone_removibile"
ref_plane "Piano di lavoro6" through (0, -13, 0) normal (0, 1, 0) x (0, 0, 1) in component "14_Guscio_mobile_cannone_removibile"
sketch "Schizzo10 (6)" plane through (0, -13, 0) normal (0, 1, 0) x (1, 0, 0) in component "14_Guscio_mobile_cannone_removibile"
  line L0 (-7, -90.5) -> (7, -90.5)
  line L1 (7, -90.5) -> (7, -109.5)
  line L2 (7, -109.5) -> (-7, -109.5)
  line L3 (-7, -109.5) -> (-7, -90.5)
extrude "Finestra_posteriore_culatta_manuale" cut sketch "Schizzo10 (6)" along normal blind 2.5 bodies 30 in component "14_Guscio_mobile_cannone_removibile"
sketch "Schizzo11 (5)" plane through (0, 0, 107) normal (0, 0, 1) x (1, 0, 0) in component "14_Guscio_mobile_cannone_removibile"
  line L0 (-7, -13) -> (7, -13)
  line L1 (7, -13) -> (7, -1)
  line L2 (7, -1) -> (-7, -1)
  line L3 (-7, -1) -> (-7, -13)
extrude "Asola_tetto_accesso_culatta_manuale" cut sketch "Schizzo11 (5)" along normal blind 2.5 bodies 30 in component "14_Guscio_mobile_cannone_removibile"